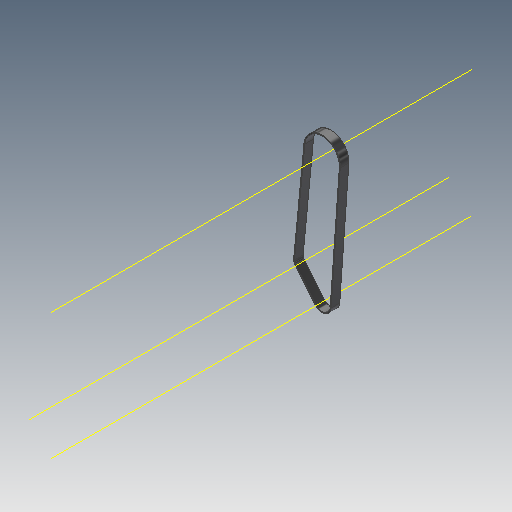
# Autodesk Inventor part: Synchronous Belt
Saved by Autodesk Inventor 2018 (Build 220112000, 112)
## iProperties
Created: 2019-08-30
Part Number: Synchronous Belt
Material: Rubber
Document SubType Name: Modeling
Designer: Clevo
Density: 1 g/cm^3
Appearance: Rubber - Black - Version 1.1
CustomPartVersion: 1
Author: Clevo
Autodesk Inventor part; units mm, degrees
sketch "Sketch Path" plane through (0, 0, 0) normal (0, 0, 1) x (1, 0, 0)
  arc A0 (-4.5858, -3.8198) -> (5.9527, -0.4318) centre (0, 0) ccw
  arc A1 (-19.4599, 15.888) -> (-18.5572, 12.9535) centre (-15.5, 15.5) ccw
  arc A2 (12.3022, 87.1077) -> (-12.2757, 89.2029) centre (0, 88) ccw
  line L0 (12.3022, 87.1077) -> (5.9527, -0.4318)
  line L1 (-4.5858, -3.8198) -> (-18.5572, 12.9535)
  line L2 (-19.4599, 15.888) -> (-12.2757, 89.2029)
  constraints: 6 end point, 4 point on circle, 2 centre point, 3 other
ref_plane "Cross Section Plane" through (5.9527, -0.4318, 0) normal (0.0723, 0.9974, 0) x (0, 0, 1)
ref_plane "Work Plane2" through (0, 0, 0) normal (-1, 0, 0) x (0, 0, 1)
ref_plane "Work Plane3" through (-15.5, 15.5, 0) normal (0.2665, -0.9638, 0) x (0, 0, 1)
ref_plane "Work Plane4" through (0, 88, 0) normal (-0.286, -0.9582, 0) x (0, 0, 1)
sketch "Cross Section" plane through (5.9527, -0.4318, 0) normal (0.0723, 0.9974, 0) x (0, 0, 1)
  line L0 (-3, 0.3) -> (3, 0.3)
  line L1 (3, 0.3) -> (3, -0.3)
  line L2 (3, -0.3) -> (-3, -0.3)
  line L3 (-3, -0.3) -> (-3, 0.3)
  line L4 (-3, 0) -> (3, 0) construction
  point P0 (0, 0)
  point P1 (0, 0)
  dimension "d0" = 6
  dimension "d4" = 0.3
  dimension "d5" = 0.3
  constraints: 10 end point, 3 midpoint, 2 parallel, 1 coincident, 1 horizontal, 1 perpendicular, 1 other
  measures "d0" distance between parallel lines of L1 L3
  measures "d4" distance between parallel lines of L2 L4
  measures "d5" distance between parallel lines of L4 L0
sweep "Belt" add profiles "Cross Section" path "Sketch Path"
equation "\"d0\" = da_B"
equation "\"d4\" = da_a"
equation "\"d5\" = da_a2"
equation "\"da_B\" = 6"
equation "\"da_pb\" = 2.5"
equation "\"da_L\" = 239.02838"
equation "\"da_a\" = 0.3"
equation "\"da_S\" = 1.5"
equation "\"da_Beta\" = 20deg"
equation "\"da_Ht\" = 0.7"
equation "\"da_H\" = 1.3"
equation "\"da_a2\" = 0.3"
body "Solid1"
